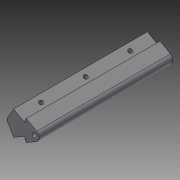
# Autodesk Inventor part: ServoHousing_alternateLaser
Saved by Autodesk Inventor 2014 SP1 (Build 180222100, 222)
## iProperties
Created: 2014-11-10
Part Number: ServoHousing_alternateLaser
Material: Generic
Document SubType Name: Modeling
Designer: rawrdong
Density: 1 g/cm^3
Appearance: Default
Author: rawrdong
Autodesk Inventor part; units mm, degrees
ref_plane "YZ Plane" through (0, 0, 0) normal (1, 0, 0) x (0, 1, 0)
ref_plane "XZ Plane" through (0, 0, 0) normal (0, 1, 0) x (-1, 0, 0)
ref_plane "XY Plane" through (0, 0, 0) normal (0, 0, 1) x (1, 0, 0)
sketch "Sketch1" plane through (0, 0, 0) normal (0, 1, 0) x (-1, 0, 0)
  circle A0 centre (0, 0) radius 3.5
  circle A1 centre (0, 0) radius 1.4
  line L0 (-1.75, 3.0311) -> (5.1782, 7.0311)
  line L1 (-1.75, -3.0311) -> (5.1782, -7.0311)
  circle A2 centre (0, 0) radius 8.7321 construction
  line L2 (5.1782, 7.0311) -> (6.7782, 4.2598)
  line L3 (5.1782, -7.0311) -> (6.7782, -4.2598)
  line L4 (6.7782, -4.2598) -> (13.7064, -8.2598)
  line L5 (13.7064, 8.2598) -> (6.7782, 4.2598)
  line L6 (0, 0) -> (22.073, 0) construction
  line L7 (28.234, 0) -> (-14.8931, 0) projected
  line L8 (13.7064, 8.2598) -> (18.4752, 0)
  line L9 (13.7064, -8.2598) -> (18.4752, 0)
  circle A3 centre (7.4918, 0) radius 1.4
  point P0 (12.2929, 0)
  dimension "d0" = 7
  dimension "d1" = 2.8
  dimension "d4" = 3.2
  dimension "d13" = 60
  dimension "d25" = 8
  dimension "d26" = 8
  constraints: 18 end point, 5 perpendicular, 4 centre point, 4 point on circle, 4 point on line, 3 coincident, 2 tangent, 1 equal radius, 2 other
  measures "d0" diameter of A0
  measures "d1" diameter of A1
  measures "d4" distance of L1.end L3.end
  measures "d13" angle of L1 L0
  measures "d25" distance from line of point (0, 0) L3
  measures "d26" distance of L3.end L4.end
extrude "Extrusion1" add sketch "Sketch1" along normal blind 90 contours L7 A1 A0 | L7 A3 L9 L4 L3 L1 A0 | A0 L7 A1 | A0 L0 L2 L5 L8 L7 A3 | A3 L7 | L7 A3
fillet "Fillet1" radius 2 1 edges at (-18.4752, 45, 0)
sketch "Sketch2" plane through (-6.7782, 0, -4.2598) normal (0.5, 0, -0.8660254) x (-0.8660254, 0, -0.5)
  line L0 (0, 0) -> (8, 0) projected
  circle A0 centre (4, 15) radius 1.4
  line L1 (8, 0) -> (8, 90) projected
  circle A1 centre (4, 45) radius 1.4
  circle A2 centre (4, 75) radius 1.4
  point P0 (-8, 0)
  point P1 (4, 0)
  point P2 (8, 45)
  dimension "d10" = 2.8
  dimension "d16" = 30
  constraints: 3 centre point, 2 midpoint, 1 horizontal alignment, 1 vertical, 1 vertical alignment, 4 other
  measures "d10" diameter of A0
  measures "d16" distance of A0.centre A1.centre
extrude "Extrusion2" cut sketch "Sketch2" against normal blind 3.35
sketch "Sketch3" plane through (0, 90, 0) normal (0, 1, 0) x (1, 0, 0)
  line L0 (-13.7064, -8.2598) -> (-6.7782, -4.2598) projected
  line L1 (-6.7782, -4.2598) -> (-5.1782, -7.0311) projected
  circle A0 centre (-6.4657, -4.8011) radius 0.625
  line L2 (-6.1532, -5.3423) -> (-6.1532, -5.3423)
  dimension "d21" = 1.25
  constraints: 2 end point, 2 point on circle, 2 point on line, 2 tangent, 1 centre point, 1 coincident, 1 perpendicular, 3 other
  measures "d21" diameter of A0
extrude "Extrusion3" cut sketch "Sketch3" against normal through all
mirror "Mirror1" about plane through (0, 0, 0) normal (0, 0, 1) of "Extrusion2", "Extrusion3"
fillet "Fillet2" radius 0.25 2 edges at (-6.1532, 45, -5.3423) (-6.1532, 45, 5.3423)
body "Solid1"
